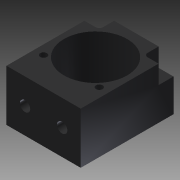
# Autodesk Inventor part: Sonar Mount
Saved by Autodesk Inventor 2015 (Build 190159000, 159)
## iProperties
Created: 2016-02-27
Part Number: Sonar Mount
Material: ABS Plastic
Document SubType Name: Modeling
Designer: James Yelland
Density: 1.06 g/cm^3
Appearance: Smooth - White
Author: James Yelland
Autodesk Inventor part; units mm, degrees
ref_plane "YZ Plane" through (0, 0, 0) normal (1, 0, 0) x (0, 1, 0)
ref_plane "XZ Plane" through (0, 0, 0) normal (0, 1, 0) x (-1, 0, 0)
ref_plane "XY Plane" through (0, 0, 0) normal (0, 0, 1) x (1, 0, 0)
sketch "Sketch1" plane through (0, 0, 0) normal (0, 1, 0) x (-1, 0, 0)
  line L0 (-10, -6.9) -> (10, -6.9)
  line L1 (10, -6.9) -> (10, 6.9)
  line L2 (10, 6.9) -> (-10, 6.9)
  line L3 (-10, 6.9) -> (-10, -6.9)
  line L4 (-10, -6.9) -> (10, 6.9) construction
  line L5 (10, -6.9) -> (-10, 6.9) construction
  point P0 (0, 0)
  dimension "d0" = 20
  dimension "d1" = 13.8
  constraints: 12 end point, 2 midpoint, 2 parallel, 1 horizontal, 1 perpendicular
  measures "d0" distance of L0.start L0.end
  measures "d1" distance of L1.end L0.end
extrude "Extrusion1" add sketch "Sketch1" along normal blind 25
sketch "Sketch2" plane through (-10, 0, 6.9) normal (0, 0, 1) x (1, 0, 0)
  circle A0 centre (10, 14) radius 8.5
  circle A1 centre (2.5, 7.5) radius 0.9
  circle A2 centre (17.5, 7.5) radius 0.9
  point P0 (10, 0)
  dimension "d14" = 17
  dimension "d18" = 1.8
  dimension "d21" = 1.8
  constraints: 3 centre point
  measures "d14" diameter of A0
  measures "d18" diameter of A1
  measures "d21" diameter of A2
extrude "Extrusion2" cut sketch "Sketch2" against normal through all contours A0
sketch "Sketch3" plane through (-10, 0, 6.9) normal (0, 0, 1) x (1, 0, 0)
  circle A0 centre (10, 14) radius 8.5
  circle A1 centre (2.5, 7.5) radius 0.9
  circle A2 centre (17.5, 7.5) radius 0.9
  point P0 (10, 0)
  point P1 (10, 0)
  dimension "d24" = 17
  dimension "d25" = 1.8
  dimension "d26" = 1.8
  constraints: 3 centre point
  measures "d24" diameter of A0
  measures "d25" diameter of A1
  measures "d26" diameter of A2
extrude "Extrusion3" cut sketch "Sketch3" against normal blind 12 contours A1 | A2
sketch "Sketch5" plane through (-10, 0, 6.9) normal (0, 0, 1) x (1, 0, 0)
  circle A0 centre (2.5, 7.5) radius 0.9 projected
  circle A1 centre (17.5, 7.5) radius 0.9 projected
  circle A2 centre (10, 14) radius 8.5 projected
  line L0 (0, 0) -> (20, 0) projected
  line L1 (20, 0) -> (20, 25) projected
  line L2 (0, 25) -> (20, 25) projected
  line L3 (0, 0) -> (0, 25) projected
  line L4 (10, 0) -> (10, 5)
  line L5 (0, 25) -> (4, 25)
  line L6 (4, 25) -> (4, 21)
  line L7 (4, 21) -> (0, 21)
  line L8 (20, 25) -> (16, 25)
  line L9 (0, 25) -> (20, 25) projected
  line L10 (16, 25) -> (16, 21)
  line L11 (16, 21) -> (20, 21)
  line L12 (20, 25) -> (20, 21)
  line L13 (20, 0) -> (20, 25) projected
  line L14 (0, 25) -> (4, 25)
  line L15 (4, 25) -> (4, 21)
  line L16 (4, 21) -> (0, 21)
  line L17 (0, 21) -> (0, 25)
  line L18 (16, 25) -> (20, 25)
  line L19 (20, 25) -> (20, 21)
  line L20 (20, 21) -> (16, 21)
  line L21 (16, 21) -> (16, 25)
  dimension "d33" = 5
  dimension "d38" = 4
  dimension "d39" = 4
  dimension "d40" = 4
  constraints: 32 end point, 6 perpendicular, 4 parallel, 3 point on line, 2 horizontal, 1 collinear, 1 vertical
  measures "d33" distance of L4.start L4.end
  measures "d38" distance of L5.end L6.end
  measures "d39" distance of L1.end L8.end
  measures "d40" distance of L8.end L10.end
extrude "Extrusion4" cut sketch "Sketch5" against normal blind 5 contours L3 L2 L6 L7 | L11 L10 L2 L1
fillet "Fillet1" radius 1 2 edges at (-6, 21, 4.4) (6, 21, 4.4)
sketch "Sketch6" plane through (0, 0, 0) normal (0, -1, 0) x (1, 0, 0)
  circle A0 centre (-5, 0) radius 1.4
  circle A1 centre (5, 0) radius 1.4
  point P0 (0, 0)
  dimension "d46" = 2.8
  dimension "d47" = 2.8
  constraints: 2 centre point
  measures "d46" diameter of A0
  measures "d47" diameter of A1
extrude "Extrusion5" cut sketch "Sketch6" against normal blind 5
body "Solid1"
